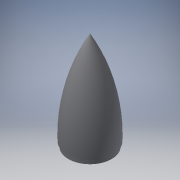
# Autodesk Inventor part: Nose Cone2
Saved by Autodesk Inventor 2019.4 (Build 234330000, 330)
## iProperties
Created: 2022-01-22
Part Number: Nose Cone2
Material: Generic
Document SubType Name: Modeling
Designer: juand
Density: 1 g/cm^3
Appearance: Default
Author: juand
Autodesk Inventor part; units mm, degrees
ref_plane "YZ Plane" through (0, 0, 0) normal (1, 0, 0) x (0, 1, 0)
ref_plane "XZ Plane" through (0, 0, 0) normal (0, 1, 0) x (-1, 0, 0)
ref_plane "XY Plane" through (0, 0, 0) normal (0, 0, 1) x (1, 0, 0)
sketch "Sketch1" plane through (0, 0, 0) normal (1, 0, 0) x (0, 1, 0)
  arc A0 (0, -34.5) -> (140, 0) centre (8.1306, 233.814) ccw
  line L0 (0, -34.5) -> (0, -32.5)
  line L1 (0, -32.5) -> (-7, -32.5)
  arc A1 (1.2, -33.3333) -> (137.5398, 0) centre (8.1306, 233.814) ccw
  line L2 (1.2, -33.3333) -> (1.2, -31.3)
  line L3 (1.2, -31.3) -> (-7, -31.3)
  line L4 (140, 0) -> (137.5398, 0)
  line L5 (185.5759, 0) -> (-49.8661, 0) construction
  line L6 (-7, -32.5) -> (-7, -31.3)
  dimension "d8" = 2
  dimension "d9" = 7
  dimension "d10" = 1.2
  constraints: 14 end point, 4 point on circle, 2 centre point, 2 horizontal, 2 perpendicular, 1 vertical, 1 other
  measures "d8" distance of L0.start L0.end
  measures "d9" distance of L0.end L1.end
  measures "d10" radial gap between concentric circles of A0 A1
revolve "Revolution2" add sketch "Sketch1" angle 360 about axis through (0, 185.5759, 0) along (0, -1, 0)
body "Solid2"
